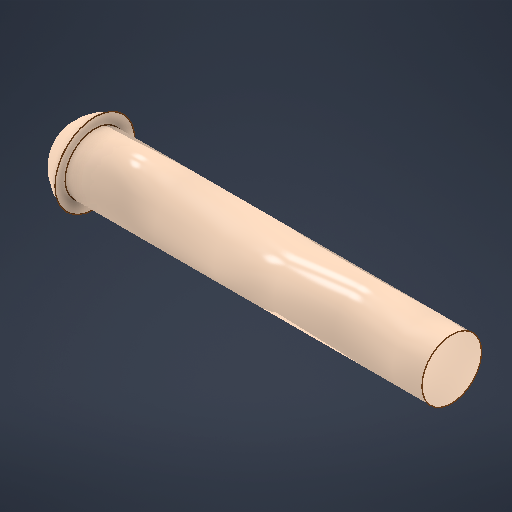
# Autodesk Inventor part: parca8
Saved by Autodesk Inventor 2025.4 (Build 294407000, 407)
## iProperties
Created: 2026-06-20
Part Number: parca8
Material: Generic
Document SubType Name: Modeling
Designer: yigithan
Density: 1 g/cm^3
Appearance: Exterior - Beige
Author: yigithan
Autodesk Inventor part; units mm, degrees
ref_plane "YZ Plane" through (0, 0, 0) normal (1, 0, 0) x (0, 1, 0)
ref_plane "XZ Plane" through (0, 0, 0) normal (0, 1, 0) x (-1, 0, 0)
ref_plane "XY Plane" through (0, 0, 0) normal (0, 0, 1) x (1, 0, 0)
sketch "Sketch1" plane through (0, 0, 0) normal (0, 0, 1) x (1, 0, 0)
  line L0 (-12.9941, 0) -> (13.2957, 0)
  line L1 (-8.4709, 1.59) -> (10.5791, 1.59)
  line L2 (-8.4709, 1.59) -> (-8.4709, 2.13)
  line L3 (-8.4709, 1.59) -> (-8.4709, 0)
  line L4 (10.5791, 1.59) -> (10.5791, 0)
  arc A0 (-8.4709, 2.13) -> (-10.3191, 0) centre (-7.507, -0.5733) ccw
  point P0 (0, 0)
  dimension "d0" = 3.18
  dimension "d1" = 19.05
  dimension "d2" = 4.26
  dimension "d3" = 2.87
  constraints: 10 end point, 3 point on line, 2 horizontal, 2 perpendicular, 2 point on circle, 1 centre point, 1 vertical
  measures "d0" diameter of L1 L0
  measures "d1" distance of L1.start L1.end
  measures "d2" diameter of L2.end L0
  measures "d3" radius of A0
revolve "Revolution1" add sketch "Sketch1" angle 360 about axis through (-12.9941, 0, 0) along (1, 0, 0)
body "Solid1"
